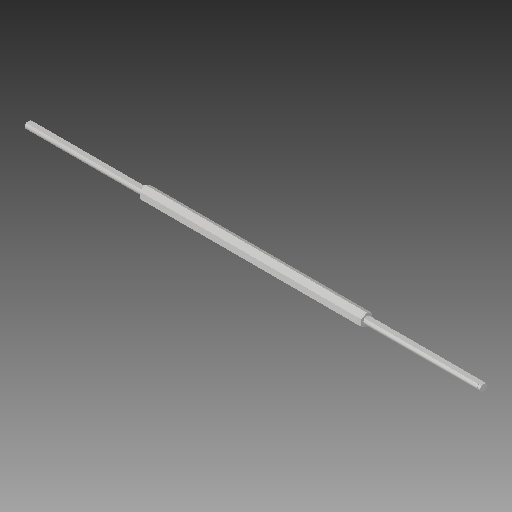
# Autodesk Inventor part: Intake Axle
Saved by Autodesk Inventor 2019.4 (Build 234330000, 330)
## iProperties
Created: 2020-01-29
Part Number: Intake Axle
Material: Aluminum 6061
Document SubType Name: Modeling
Designer: admin
Density: 2.7 g/cm^3
Appearance: Aluminum - Flat
Mass: 118.941 g
Surface Area: 179.656 cm^2
Volume: 44.0522 cm^3
Author: admin
Autodesk Inventor part; units mm, degrees
ref_plane "YZ Plane" through (0, 0, 0) normal (1, 0, 0) x (0, 1, 0)
ref_plane "XZ Plane" through (0, 0, 0) normal (0, 1, 0) x (-1, 0, 0)
ref_plane "XY Plane" through (0, 0, 0) normal (0, 0, 1) x (1, 0, 0)
sketch "Sketch1" plane through (0, 0, 0) normal (0, 0, 1) x (1, 0, 0)
  line L0 (0, 0) -> (0, 4)
  line L1 (129.5, 4) -> (129.5, 8)
  line L2 (129.5, 8) -> (375.7, 8)
  line L3 (375.7, 8) -> (375.7, 4)
  line L4 (505.2, 4) -> (505.2, 0)
  line L5 (505.2, 0) -> (0, 0)
  line L6 (375.7, 4) -> (382.6, 4)
  line L7 (382.6, 4) -> (382.6, 3.65)
  line L8 (382.6, 3.65) -> (383.7, 3.65)
  line L9 (383.7, 3.65) -> (383.7, 4)
  line L10 (383.7, 4) -> (399.7, 4)
  line L11 (399.7, 4) -> (399.7, 3.65)
  line L12 (399.7, 3.65) -> (400.8, 3.65)
  line L13 (400.8, 3.65) -> (400.8, 4)
  line L14 (400.8, 4) -> (505.2, 4)
  line L15 (129.5, 4) -> (0, 4)
  dimension "d2" = 246.2
  dimension "d3" = 8
  dimension "d4" = 129.5
  dimension "d5" = 129.5
  dimension "d6" = 1.1
  dimension "d7" = 1.1
  dimension "d8" = 0.35
  dimension "d11" = 4
  dimension "d12" = 4
  dimension "d13" = 8
  dimension "d14" = 16
  constraints: 32 end point, 9 perpendicular, 5 point on line, 2 horizontal, 1 vertical
  measures "d2" distance of L1.end L2.end
  measures "d3" distance between parallel lines of L5 L2
  measures "d4" distance of L0.end L1.start
  measures "d5" distance of L3.end L4.start
  measures "d6" distance of L7.end L8.end
  measures "d7" distance of L11.end L12.end
  measures "d8" distance of L6.end L7.end
  measures "d11" distance between parallel lines of L5 L15
  measures "d12" distance between parallel lines of L5 L14
  measures "d13" distance between parallel lines of L3 L9
  measures "d14" distance of L9.end L10.end
revolve "Revolution1" add sketch "Sketch1" angle 360 about axis through (505.2, 0, 0) along (-1, 0, 0)
sketch "Sketch2" plane through (375.7, 0, 0) normal (1, 0, 0) x (0, 0, -1)
  circle A0 centre (0, 0) radius 8 projected
  line L0 (0, 7.1014) -> (6.15, 3.5507)
  line L1 (6.15, 3.5507) -> (6.15, -3.5507)
  line L2 (6.15, -3.5507) -> (0, -7.1014)
  line L3 (0, -7.1014) -> (-6.15, -3.5507)
  line L4 (-6.15, -3.5507) -> (-6.15, 3.5507)
  line L5 (-6.15, 3.5507) -> (0, 7.1014)
  point P0 (0, 0)
  dimension "d16" = 12.3
  constraints: 12 end point, 1 coincident, 13 other
  measures "d16" distance between parallel lines of L4 L1
extrude "Extrusion1" cut sketch "Sketch2" against normal up to surface (246.2 mm away)
sketch "Sketch3" plane through (400.8, 0, 0) normal (1, 0, 0) x (0, 0, -1)
  line L0 (-2.6458, 3) -> (2.6458, 3)
  circle A0 centre (0, 0) radius 4 projected
  point P0 (0, 0)
  dimension "d19" = 3
  constraints: 2 end point, 2 point on circle, 1 horizontal
  measures "d19" distance from line of A0.centre L0
extrude "Extrusion2" cut sketch "Sketch3" against normal up to surface (18.2 mm away) contours A0 L0 picked at (-0.6179, 3.1815)
sketch "Sketch4" plane through (505.2, 0, 0) normal (1, 0, 0) x (0, 0, -1)
  circle A0 centre (0, 0) radius 4 projected
  line L0 (-2.6458, 3) -> (2.6458, 3)
  dimension "d31" = 3
  constraints: 2 end point, 2 point on circle, 1 horizontal
  measures "d31" distance from line of L0 A0.centre
extrude "Extrusion3" cut sketch "Sketch4" against normal blind 165.3 contours L0 A0 picked at (-0.6179, 3.1815)
ref_plane "Work Plane1" through (503.2, 3.8, 2.1939) normal (1, 0, 0) x (0, 0, -1)
sketch "Sketch5" plane through (503.2, 3.8, 2.1939) normal (1, 0, 0) x (0, 0, -1)
  circle A0 centre (2.1939, -3.8) radius 4 projected
  circle A1 centre (2.1939, -3.8) radius 3.75
  dimension "d32" = 7.5
  constraints: 1 centre point, 1 coincident
  measures "d32" diameter of A1
extrude "Extrusion4" cut sketch "Sketch5" against normal blind 1.1
ref_plane "Work Plane2" through (252.6, -3.5507, -6.15) normal (1, 0, 0) x (0, 0, -1)
mirror "Mirror1" about plane through (252.6, -3.5507, -6.15) normal (1, 0, 0) of "Extrusion3", "Extrusion4"
body "Solid1"
